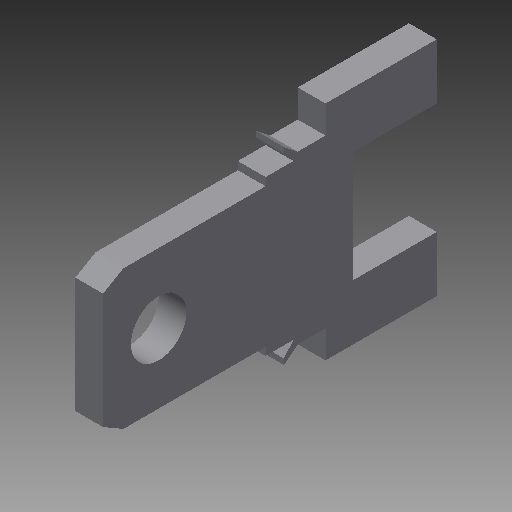
# Autodesk Inventor part: Polo2
Saved by Autodesk Inventor 2017 (Build 210142000, 142)
## iProperties
Created: 2016-05-14
Part Number: Polo2
Material: Genérico
Document SubType Name: Modeling
Designer: Isra
Density: 1 g/cm^3
Appearance: Valor por defecto
Author: Isra
Autodesk Inventor part; units mm, degrees
ref_plane "YZ Plane" through (0, 0, 0) normal (1, 0, 0) x (0, 1, 0)
ref_plane "XZ Plane" through (0, 0, 0) normal (0, 1, 0) x (-1, 0, 0)
ref_plane "XY Plane" through (0, 0, 0) normal (0, 0, 1) x (1, 0, 0)
sketch "Boceto1" plane through (0, 0, 0) normal (0, 0, 1) x (1, 0, 0)
  line L0 (0.5, -3) -> (-0.5, -3)
  line L1 (-0.5, -3) -> (-0.5, 3)
  line L2 (-0.5, 3) -> (0.5, 3)
  line L3 (0.5, 3) -> (0.5, -3)
  line L4 (0.5, -3) -> (-0.5, 3) construction
  line L5 (-0.5, -3) -> (0.5, 3) construction
  point P0 (0, 0)
  dimension "d0" = 1
  dimension "d1" = 6
  constraints: 12 end point, 2 midpoint, 2 parallel, 1 horizontal, 1 perpendicular
  measures "d0" distance of L1.end L2.end
  measures "d1" distance of L0.end L1.end
sketch "Boceto2" plane through (0, 0, 0) normal (1, 0, 0) x (0, 1, 0)
  line L0 (0, 0) -> (0, 7)
  line L1 (2.5, 1.1547) -> (2.5, 6.2702)
  line L2 (2.5, 6.2702) -> (2.0787, 7)
  line L3 (2.0787, 7) -> (0, 7)
  line L4 (2.5, 1.1547) -> (2.6776, 1.1547)
  line L5 (2.6776, 1.1547) -> (2.7854, 1.1547)
  line L6 (2.7854, 1.1547) -> (2.7854, 0.1547)
  line L7 (2.7854, 0.1547) -> (3.1939, 0.4965)
  line L8 (3.1939, 0.4965) -> (3.3939, 0.4965)
  line L9 (3.3939, 0.4965) -> (3, 0)
  line L10 (-2.5, 1.1547) -> (-2.5, 6.2702)
  line L11 (-2.5, 6.2702) -> (-2.0787, 7)
  line L12 (-2.0787, 7) -> (0, 7)
  line L13 (-2.5, 1.1547) -> (-2.6776, 1.1547)
  line L14 (-2.6776, 1.1547) -> (-2.7854, 1.1547)
  line L15 (-2.7854, 1.1547) -> (-2.7854, 0.1547)
  line L16 (-2.7854, 0.1547) -> (-3.1939, 0.4965)
  line L17 (-3.1939, 0.4965) -> (-3.3939, 0.4965)
  line L18 (-3.3939, 0.4965) -> (-3, 0)
  line L19 (3, 0) -> (-3, 0)
  circle A0 centre (0, 5) radius 1
  dimension "d2" = 7
  dimension "d3" = 120
  dimension "d8" = 0.2
  dimension "d9" = 1
  dimension "d10" = 2
  dimension "d11" = 2
  constraints: 42 end point, 11 symmetric about line, 3 horizontal, 3 point on line, 2 vertical, 1 centre point, 1 perpendicular
  measures "d2" distance of L0.start L0.end
  measures "d3" angle of L3 L2
  measures "d8" distance of L7.end L8.end
  measures "d9" distance of L5.end L6.end
  measures "d10" diameter of A0
  measures "d11" distance from line of L3 A0.centre
extrude "Extrusión1" add sketch "Boceto2" along normal mid plane 1 contours L19 L18 L17 L16 L15 L14 L13 L10 L11 L12 L0 A0 | L0 A0 L3 L2 L1 L4 L5 L6 L7 L8 L9 L19
extrude "Extrusión2" add sketch "Boceto1" against normal blind 1
sketch "Boceto3" plane through (0, 0, -1) normal (0, 0, -1) x (-1, 0, 0)
  line L0 (-0.5, 4) -> (0.5, 4)
  line L1 (0.5, 4) -> (0.5, -4)
  line L2 (0.5, -4) -> (-0.5, -4)
  line L3 (-0.5, -4) -> (-0.5, 4)
  line L4 (-0.5, 4) -> (0.5, -4) construction
  line L5 (0.5, 4) -> (-0.5, -4) construction
  line L6 (-0.5, 2) -> (0.5, 2)
  line L7 (0.5, 2) -> (0.5, -2)
  line L8 (0.5, -2) -> (-0.5, -2)
  line L9 (-0.5, -2) -> (-0.5, 2)
  line L10 (-0.5, 2) -> (0.5, -2) construction
  line L11 (0.5, 2) -> (-0.5, -2) construction
  point P0 (0, 0)
  dimension "d16" = 8
  dimension "d17" = 4
  constraints: 24 end point, 4 midpoint, 4 parallel, 2 horizontal, 2 perpendicular, 1 point on line
  measures "d16" distance of L0.end L1.end
  measures "d17" distance of L6.end L7.end
extrude "Extrusión3" add sketch "Boceto3" along normal blind 4 contours L0 L1 L6 L3 | L8 L1 L2 L3
sketch "Boceto4" plane through (0, 0, -1) normal (0, 0, -1) x (-1, 0, 0)
  line L0 (-0.5, 2) -> (0.5, 2)
  line L1 (0.5, 2) -> (0.5, -2)
  line L2 (0.5, -2) -> (-0.5, -2)
  line L3 (-0.5, -2) -> (-0.5, 2)
  line L4 (-0.5, 2) -> (0.5, -2) construction
  line L5 (0.5, 2) -> (-0.5, -2) construction
  point P0 (0, 0)
  dimension "d20" = 1
  dimension "d21" = 4
  constraints: 12 end point, 2 midpoint, 2 parallel, 1 horizontal, 1 perpendicular
  measures "d20" distance of L1.end L2.end
  measures "d21" distance of L0.end L1.end
extrude "Extrusión4" add sketch "Boceto4" along normal blind 1
